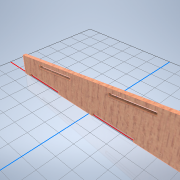
# Autodesk Inventor part: ControlPanelSide_V1
Saved by Autodesk Inventor 2022.2 (Build 262287000, 287)
## iProperties
Created: 2022-11-16
Part Number: ControlPanelSide_V1
Material: Generic
Document SubType Name: Modeling
Designer: jaege
Density: 1 g/cm^3
Appearance: Red Oak - Natural Low Gloss
Author: jaege
Autodesk Inventor part; units mm, degrees
ref_plane "YZ Plane" through (0, 0, 0) normal (1, 0, 0) x (0, 1, 0)
ref_plane "XZ Plane" through (0, 0, 0) normal (0, 1, 0) x (-1, 0, 0)
ref_plane "XY Plane" through (0, 0, 0) normal (0, 0, 1) x (1, 0, 0)
sketch "Sketch2" plane through (0, 0, 0) normal (0, 1, 0) x (-1, 0, 0)
  line L0 (105, -2) -> (-105, -2)
  line L1 (-105, -2) -> (-105, 2)
  line L2 (-105, 2) -> (105, 2)
  line L3 (105, 2) -> (105, -2)
  line L4 (105, -2) -> (-105, 2) construction
  line L5 (-105, -2) -> (105, 2) construction
  point P0 (0, 0)
  dimension "d1" = 210
  dimension "d2" = 4
  constraints: 12 end point, 2 midpoint, 2 parallel, 1 horizontal, 1 perpendicular
  measures "d1" distance of L1.end L2.end
  measures "d2" distance of L0.end L1.end
extrude "Extrusion1" add sketch "Sketch2" along normal blind 100
sketch "Sketch3" plane through (-105, 0, 2) normal (0, 0, 1) x (1, 0, 0)
  line L0 (0, 0) -> (0, 100) projected
  line L1 (0, 20) -> (210, 50)
  line L2 (210, 0) -> (210, 100) projected
  line L3 (0, 0) -> (210, 0) projected
  line L4 (0, 0) -> (210, 0) projected
  line L5 (210, 0) -> (210, 100) projected
  line L6 (0, 100) -> (210, 100) projected
  line L7 (0, 0) -> (0, 100) projected
  point P0 (105, 0)
  dimension "d5" = 20
  dimension "d37" = 30
  constraints: 2 end point, 1 midpoint, 1 point on line
  measures "d5" distance from line of L3 L1.start
  measures "d37" vertical distance of L1.start L1.end
extrude "Extrusion2" cut sketch "Sketch3" against normal up to next contours L0 L6 L2 L1
sketch "Sketch4" plane through (0, 0, 0) normal (0, -1, 0) x (1, 0, 0)
  line L0 (105, 2) -> (55, 2)
  line L1 (55, 2) -> (55, -2)
  line L2 (55, -2) -> (105, -2)
  line L3 (105, -2) -> (105, 2)
  line L4 (-105, 2) -> (105, 2) projected
  line L5 (-105, -2) -> (-105, 2) projected
  line L6 (105, -2) -> (-105, -2) projected
  line L7 (105, 2) -> (105, -2) projected
  line L8 (55, 2) -> (5, 2)
  line L9 (5, 2) -> (5, -2)
  line L10 (5, -2) -> (55, -2)
  line L11 (55, -2) -> (55, 2)
  line L12 (5, 2) -> (-45, 2)
  line L13 (-45, 2) -> (-45, -2)
  line L14 (-45, -2) -> (5, -2)
  line L15 (5, -2) -> (5, 2)
  line L16 (-45, 2) -> (-95, 2)
  line L17 (-95, 2) -> (-95, -2)
  line L18 (-95, -2) -> (-45, -2)
  line L19 (-45, -2) -> (-45, 2)
  point P0 (0, 0)
  point P1 (55, -2)
  point P2 (5, -2)
  point P3 (-45, -2)
  dimension "d9" = 50
  dimension "d10" = 4
  dimension "d13" = 50
  constraints: 32 end point, 2 horizontal, 2 parallel, 1 perpendicular, 27 other
  measures "d9" distance of L2.end L1.end
  measures "d10" distance of L1.end L0.end
  measures "d13" distance of L1.end L9.end
extrude "Extrusion3" add sketch "Sketch4" along normal blind 4 contours L3 L2 L1 L0 | L9 L6 L13 L4 | L17 L6 L5 L4
sketch "Sketch5" plane through (-95, 0, 2) normal (0, 0, 1) x (1, 0, 0)
  line L0 (-10, 20) -> (-10, -4) projected
  line L1 (0, -4) -> (-10, -4) projected
  line L2 (0, 0) -> (0, -4) projected
  line L3 (0, 0) -> (50, 0) projected
  line L4 (50, 0) -> (50, -4) projected
  line L5 (100, -4) -> (50, -4) projected
  line L6 (100, 0) -> (100, -4) projected
  line L7 (100, 0) -> (150, 0) projected
  line L8 (150, 0) -> (150, -4) projected
  line L9 (200, -4) -> (150, -4) projected
  line L10 (200, -4) -> (200, 50) projected
  line L11 (200, 50) -> (-10, 20) projected
  line L12 (-5, 15.6635) -> (192.9899, 43.9478)
  line L13 (19.7487, 19.1991) -> (69.2462, 26.2701)
  line L14 (69.2462, 26.2701) -> (69.8119, 22.3103)
  line L15 (69.8119, 22.3103) -> (20.3144, 15.2393)
  line L16 (20.3144, 15.2393) -> (19.7487, 19.1991)
  line L17 (118.7437, 33.3412) -> (119.3094, 29.3814)
  line L18 (69.8119, 22.3103) -> (69.2462, 26.2701)
  line L19 (119.3094, 29.3814) -> (69.8119, 22.3103)
  line L20 (69.2462, 26.2701) -> (118.7437, 33.3412)
  line L21 (168.2412, 40.4123) -> (168.8068, 36.4525)
  line L22 (119.3094, 29.3814) -> (118.7437, 33.3412)
  line L23 (168.8068, 36.4525) -> (119.3094, 29.3814)
  line L24 (118.7437, 33.3412) -> (168.2412, 40.4123)
  line L25 (200, 50) -> (-10, 20) projected
  point P0 (95, 0)
  point P1 (200, 100)
  point P2 (168.2412, 40.4123)
  dimension "d20" = 200
  dimension "d24" = 4
  dimension "d25" = 50
  dimension "d26" = 5
  dimension "d27" = 25
  dimension "d30" = 50
  constraints: 26 end point, 2 parallel, 2 point on line, 1 perpendicular, 19 other
  measures "d20" distance of L12.start L12.end
  measures "d24" distance of L13.end L14.end
  measures "d25" distance of L14.end L15.end
  measures "d26" distance from line of L0 L12.start
  measures "d27" distance of L12.start L13.start
  measures "d30" distance of L14.end L17.end
extrude "Extrusion4" cut sketch "Sketch5" against normal up to next contours L12 L14 L15 L16 | L12 L21 L23 L17
body "Solid2"
